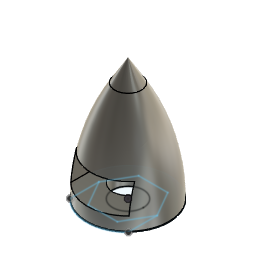
pin (Autodesk Fusion 360 design; units mm, degrees)
Autodesk Fusion 360 part; units mm, degrees
sketch "Sketch1" plane through (0, 0, 0) normal (0, 1, 0) x (1, 0, 0)
  line L0 (0, 0) -> (6, 0)
  line L1 (6, 0) -> (6, -8)
  line L2 (0, 0) -> (0, -18)
  line L3 (0, -18) -> (6, -8)
  dimension "d1" = 6
  dimension "d2" = 8
  dimension "d3" = 18
  constraint coincident L0.start L2.start
  constraint horizontal L0
  constraint perpendicular L0 L1
  constraint perpendicular L0 L2
  measures "d1" distance of L0.start L0.end
  measures "d2" distance of L0.end L1.end
  measures "d3" distance of L0.start L2.end
revolve "Revolve1" add sketch "Sketch1" angle 360 about axis through (0, 0, 0) along (0, 0, 1)
sketch "Sketch2" plane through (0, 0, 0) normal (0, 0, -1) x (1, 0, 0)
  circle A0 centre (0, 0) radius 6
  line L0 (2.1362, -3.7) -> (4.2724, 0)
  line L1 (4.2724, 0) -> (2.1362, 3.7)
  line L2 (2.1362, 3.7) -> (-2.1362, 3.7)
  line L3 (-2.1362, 3.7) -> (-4.2724, 0)
  line L4 (-4.2724, 0) -> (-2.1362, -3.7)
  line L5 (-2.1362, -3.7) -> (2.1362, -3.7)
  line L6 (-4.2724, 0) -> (-4.2724, 4.2127)
  line L7 (4.2724, 0) -> (4.2724, 4.2127)
  arc A1 (4.2724, 4.2127) -> (-4.2724, 4.2127) centre (0, 0) ccw
  circle A2 centre (0, 0) radius 2.25
  dimension "d5" = 3.7
  dimension "d6" = 180
  dimension "d10" = 4.5
  constraint coincident A0.centre A1.centre
  constraint vertical L6
  constraint coincident A0 L6.end
  constraint coincident A0 L7.end
  measures "d5" distance of A0.centre L5
  measures "d6" angle of L6 L7
  measures "d10" diameter of A2
extrude "Extrude2" cut sketch "Sketch2" against normal blind 10 contours A2
extrude "Extrude1" cut sketch "Sketch2" against normal blind 4 from surface at -2 contours A0 L1 L2 L3 L6 L7 A1 | L0 L1 L2 L3 L4 L5 | A2
fillet "Fillet1" radius 28.5 1 faces at (-1.8267, -4.6544, 9.6667)
